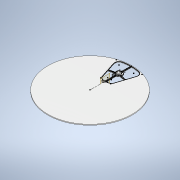
# Autodesk Inventor part: StatorSketches
Saved by Autodesk Inventor 2022.2 (Build 262287000, 287)
## iProperties
Created: 2022-08-10
Part Number: StatorSketches
Material: ABS Plastic
Document SubType Name: Modeling
Designer: ABL
Density: 1.06 g/cm^3
Appearance: Smooth - White
Author: ABL
Autodesk Inventor part; units mm, degrees
ref_plane "YZ Plane" through (0, 0, 0) normal (1, 0, 0) x (0, 1, 0)
ref_plane "XZ Plane" through (0, 0, 0) normal (0, 1, 0) x (-1, 0, 0)
ref_plane "XY Plane" through (0, 0, 0) normal (0, 0, 1) x (1, 0, 0)
sketch "SpoolBorder" plane through (0, 0, 0) normal (0, 0, 1) x (1, 0, 0)
  line L0 (13.9597, -42.9634) -> (26.7564, -82.3478)
  line L1 (0, 0) -> (0, -97.1611) construction
  arc A0 (0, -97.1611) -> (19.2245, -95.2402) centre (0, 0) ccw
  arc A1 (5.3164, -36.0913) -> (0, -35.8603) centre (0, -97.1611) ccw
  arc A2 (19.2245, -95.2402) -> (26.7564, -82.3478) centre (17.2459, -85.4379) ccw
  arc A3 (13.9597, -42.9634) -> (5.3164, -36.0913) centre (4.4491, -46.0536) ccw
  arc A4 (-19.2245, -95.2402) -> (0, -97.1611) centre (0, 0) ccw
  arc A5 (0, -35.8603) -> (-5.3164, -36.0913) centre (0, -97.1611) ccw
  line L2 (-13.9597, -42.9634) -> (-26.7564, -82.3478)
  arc A6 (-26.7564, -82.3478) -> (-19.2245, -95.2402) centre (-17.2459, -85.4379) ccw
  arc A7 (-5.3164, -36.0913) -> (-13.9597, -42.9634) centre (-4.4491, -46.0536) ccw
  point P0 (21.032, -64.73)
  point P1 (30.0244, -92.4057)
  point P2 (12.0397, -37.0542)
  point P3 (-30.0244, -92.4057)
  point P4 (-12.0397, -37.0542)
  dimension "d6" = 97.1611
  dimension "d7" = 10
  dimension "d8" = 10
  dimension "d18" = 61.3008
  dimension "d34" = 10
  measures "d6" distance of L1.start L1.end
  measures "d7" radius of A2
  measures "d8" radius of A3
  measures "d18" distance of L1.end A1.end
  measures "d34" radius of A6
sketch "StatorSpider" plane through (0, 0, 0) normal (0, 0, 1) x (1, 0, 0)
  line L0 (0.0009, -38.9369) -> (0.0009, -97.1369) construction
  line L1 (-3.3991, -69.9999) -> (0.0009, -64.1109) construction
  line L2 (0.0009, -64.1109) -> (3.4009, -69.9999) construction
  line L3 (3.4009, -69.9999) -> (-3.3991, -69.9999) construction
  line L4 (0.0009, -64.1109) -> (3.4997, -62.0909) construction
  arc A0 (3.4997, -62.0909) -> (0.0009, -60.0709) centre (0.0009, -64.1109) ccw
  line L5 (3.4997, -62.0909) -> (6.8997, -67.9799)
  arc A1 (3.4009, -74.0399) -> (6.8997, -67.9799) centre (3.4009, -69.9999) ccw
  line L6 (3.4009, -69.9999) -> (3.4009, -74.0399) construction
  line L7 (3.4009, -69.9999) -> (6.8997, -67.9799) construction
  circle A2 centre (0.0009, -68.0369) radius 4.04
  circle A3 centre (0.0009, -68.0369) radius 1.4 construction
  line L8 (0.0009, -97.1369) -> (0.0009, -35.8361) construction
  line L9 (4.6997, -64.1694) -> (5.6997, -65.9014) construction
  line L10 (3.4009, -74.0399) -> (-3.3991, -74.0399)
  arc A4 (0.0009, -60.0709) -> (-3.4978, -62.0909) centre (0.0009, -64.1109) ccw
  line L11 (0.0009, -64.1109) -> (-3.4978, -62.0909) construction
  line L12 (0.0009, -64.1109) -> (0.0009, -60.0709) construction
  line L13 (-3.4978, -62.0909) -> (-6.8978, -67.9799)
  arc A5 (-6.8978, -67.9799) -> (-3.3991, -74.0399) centre (-3.3991, -69.9999) ccw
  point P0 (1.8944, -62.2189)
  point P1 (0.0009, -69.9999)
  point P2 (5.1997, -65.0354)
  dimension "d11" = 6.8
  dimension "d12" = 4.04
  dimension "d14" = 6.8
  dimension "d15" = 120
  dimension "d16" = 8.08
  dimension "d17" = 2.8
  dimension "d19" = 61.3008
  dimension "d24" = 2
  dimension "d35" = 6.8
  dimension "d36" = 60
  dimension "d37" = 6.8
  measures "d11" distance of L2.end L1.start
  measures "d12" distance of L1.end L4.end
  measures "d14" distance of L4.end L5.end
  measures "d15" angle of L6 L7
  measures "d16" diameter of A2
  measures "d17" diameter of A3
  measures "d19" distance of L0.end L8.end
  measures "d24" distance of L9.start L9.end
  measures "d35" distance of L6.end L10.end
  measures "d36" angle of L12 L11
  measures "d37" distance of L11.end L13.end
sketch "Sketch1" plane through (0, 0, 0) normal (0, 1, 0) x (-1, 0, 0)
  circle A0 centre (0, 0) radius 97.1611
  line L0 (0, 0) -> (0, -99.1611) construction
  circle A1 centre (0, 0) radius 38.9611 construction
  line L1 (0, 0) -> (97.1611, 0) construction
  line L2 (0, 0) -> (33.2311, -91.3016) construction
  line L3 (0, 0) -> (30.0244, -92.4057) construction
  circle A2 centre (0, 0) radius 34.9611 construction
  line L4 (0, -35.8603) -> (11.6517, -35.8603) construction
  line L5 (11.6517, -35.8603) -> (30.0244, -92.4057) construction
  circle A3 centre (0, 0) radius 99.1611
  line L6 (0, 0) -> (-30.0244, -92.4057) construction
  line L7 (0, 0) -> (-33.2311, -91.3016) construction
  line L8 (0, -35.8603) -> (-11.6517, -35.8603) construction
  line L9 (13.9597, -42.9634) -> (26.7564, -82.3478)
  line L10 (0, 0) -> (0, -97.1611) construction
  arc A4 (0, -97.1611) -> (19.2245, -95.2402) centre (0, 0) ccw
  arc A5 (5.3164, -36.0913) -> (0, -35.8603) centre (0, -97.1611) ccw
  arc A6 (19.2245, -95.2402) -> (26.7564, -82.3478) centre (17.2459, -85.4379) ccw
  arc A7 (13.9597, -42.9634) -> (5.3164, -36.0913) centre (4.4491, -46.0536) ccw
  arc A8 (-19.2245, -95.2402) -> (0, -97.1611) centre (0, 0) ccw
  arc A9 (0, -35.8603) -> (-5.3164, -36.0913) centre (0, -97.1611) ccw
  line L11 (-13.9597, -42.9634) -> (-26.7564, -82.3478)
  arc A10 (-26.7564, -82.3478) -> (-19.2245, -95.2402) centre (-17.2459, -85.4379) ccw
  arc A11 (-5.3164, -36.0913) -> (-13.9597, -42.9634) centre (-4.4491, -46.0536) ccw
  line L12 (0, -38.9611) -> (0, -97.1611) construction
  line L13 (-3.4, -70.0241) -> (0, -64.1351) construction
  line L14 (0, -64.1351) -> (3.4, -70.0241) construction
  line L15 (3.4, -70.0241) -> (-3.4, -70.0241) construction
  line L16 (0, -64.1351) -> (3.4987, -62.1151) construction
  arc A12 (3.4987, -62.1151) -> (0, -60.0951) centre (0, -64.1351) ccw
  line L17 (3.4987, -62.1151) -> (6.8987, -68.0041)
  arc A13 (3.4, -74.0641) -> (6.8987, -68.0041) centre (3.4, -70.0241) ccw
  line L18 (3.4, -70.0241) -> (3.4, -74.0641) construction
  line L19 (3.4, -70.0241) -> (6.8987, -68.0041) construction
  circle A14 centre (0, -68.0611) radius 4.04
  circle A15 centre (0, -68.0611) radius 1.4 construction
  line L20 (0, -97.1611) -> (0, -35.8603) construction
  line L21 (4.6987, -64.1936) -> (5.6987, -65.9257) construction
  line L22 (3.4, -74.0641) -> (-3.4, -74.0641)
  arc A16 (0, -60.0951) -> (-3.4987, -62.1151) centre (0, -64.1351) ccw
  line L23 (0, -64.1351) -> (-3.4987, -62.1151) construction
  line L24 (0, -64.1351) -> (0, -60.0951) construction
  line L25 (-3.4987, -62.1151) -> (-6.8987, -68.0041)
  arc A17 (-6.8987, -68.0041) -> (-3.4, -74.0641) centre (-3.4, -70.0241) ccw
  dimension "d0" = 194.3223
  dimension "d1" = 99.1611
  dimension "d2" = 77.9223
  dimension "d3" = 70
  dimension "d4" = 72
  dimension "d5" = 69.9223
  dimension "d29" = 198.3223
  dimension "d32" = 40
  dimension "d33" = 36
  constraints: 18 end point, 5 point on circle, 4 centre point, 4 coincident, 2 horizontal, 2 point on line, 1 perpendicular, 1 vertical, 5 other
  measures "d0" diameter of A0
  measures "d1" distance of L0.start L0.end
  measures "d2" diameter of A1
  measures "d3" angle of L2 L1
  measures "d4" angle of L1 L3
  measures "d5" diameter of A2
  measures "d29" diameter of A3
  measures "d32" angle of L7 L2
  measures "d33" angle of L3 L6
sketch "Sketch2" plane through (0, 0, 0) normal (0, 1, 0) x (-1, 0, 0)
  line L0 (0, 0) -> (0, -97.1611) construction
  line L1 (0, -35.8603) -> (0, -60.0951) construction
  line L2 (0, -97.1611) -> (0, -74.0641) construction
  line L3 (5.1987, -65.0596) -> (6.8987, -68.0041) construction
  line L4 (4.6987, -64.1936) -> (-4.6987, -64.1936) construction
  line L5 (5.6987, -65.9257) -> (-5.6987, -65.9257) construction
  line L6 (0, -35.8603) -> (-1, -35.8603) construction
  line L7 (-1, -35.8603) -> (-1, -35.8685) construction
  line L8 (0, -60.0951) -> (-1, -60.0951) construction
  line L9 (-1, -60.0951) -> (-1, -60.2209) construction
  line L10 (-1, -35.8685) -> (-1, -60.2209)
  line L11 (0, -60.0951) -> (1, -60.0951) construction
  line L12 (1, -60.0951) -> (1, -60.2209) construction
  line L13 (0, -35.8603) -> (1, -35.8603) construction
  line L14 (1, -35.8603) -> (1, -35.8685) construction
  line L15 (1, -35.8685) -> (1, -60.2209)
  line L16 (-1, -74.0641) -> (-1, -97.156)
  line L17 (1, -74.0641) -> (1, -97.156)
  arc A0 (4.6987, -64.1936) -> (19.89, -61.2151) centre (0, 0) ccw
  arc A1 (5.6987, -65.9257) -> (20.4481, -62.9328) centre (0, 0) ccw
  arc A2 (-19.89, -61.2151) -> (-4.6987, -64.1936) centre (0, 0) ccw
  arc A3 (-20.4481, -62.9328) -> (-5.6987, -65.9257) centre (0, 0) ccw
  line L18 (13.9597, -42.9634) -> (26.7564, -82.3478)
  line L19 (0, 0) -> (0, -97.1611) construction
  arc A4 (0, -97.1611) -> (19.2245, -95.2402) centre (0, 0) ccw
  arc A5 (5.3164, -36.0913) -> (0, -35.8603) centre (0, -97.1611) ccw
  arc A6 (19.2245, -95.2402) -> (26.7564, -82.3478) centre (17.2459, -85.4379) ccw
  arc A7 (13.9597, -42.9634) -> (5.3164, -36.0913) centre (4.4491, -46.0536) ccw
  arc A8 (-19.2245, -95.2402) -> (0, -97.1611) centre (0, 0) ccw
  arc A9 (0, -35.8603) -> (-5.3164, -36.0913) centre (0, -97.1611) ccw
  line L20 (-13.9597, -42.9634) -> (-26.7564, -82.3478)
  arc A10 (-26.7564, -82.3478) -> (-19.2245, -95.2402) centre (-17.2459, -85.4379) ccw
  arc A11 (-5.3164, -36.0913) -> (-13.9597, -42.9634) centre (-4.4491, -46.0536) ccw
  line L21 (0, -38.9611) -> (0, -97.1611) construction
  line L22 (-3.4, -70.0241) -> (0, -64.1351) construction
  line L23 (0, -64.1351) -> (3.4, -70.0241) construction
  line L24 (3.4, -70.0241) -> (-3.4, -70.0241) construction
  line L25 (0, -64.1351) -> (3.4987, -62.1151) construction
  arc A12 (3.4987, -62.1151) -> (0, -60.0951) centre (0, -64.1351) ccw
  line L26 (3.4987, -62.1151) -> (6.8987, -68.0041)
  arc A13 (3.4, -74.0641) -> (6.8987, -68.0041) centre (3.4, -70.0241) ccw
  line L27 (3.4, -70.0241) -> (3.4, -74.0641) construction
  line L28 (3.4, -70.0241) -> (6.8987, -68.0041) construction
  circle A14 centre (0, -68.0611) radius 4.04
  circle A15 centre (0, -68.0611) radius 1.4 construction
  line L29 (0, -97.1611) -> (0, -35.8603) construction
  line L30 (4.6987, -64.1936) -> (5.6987, -65.9257) construction
  line L31 (3.4, -74.0641) -> (-3.4, -74.0641)
  arc A16 (0, -60.0951) -> (-3.4987, -62.1151) centre (0, -64.1351) ccw
  line L32 (0, -64.1351) -> (-3.4987, -62.1151) construction
  line L33 (0, -64.1351) -> (0, -60.0951) construction
  line L34 (-3.4987, -62.1151) -> (-6.8987, -68.0041)
  arc A17 (-6.8987, -68.0041) -> (-3.4, -74.0641) centre (-3.4, -70.0241) ccw
  point P0 (-20.4481, -62.9328)
  point P1 (-5.6987, -65.9257)
  point P2 (-4.6987, -64.1936)
  point P3 (5.6987, -65.9257)
  point P4 (20.4481, -62.9328)
  point P5 (19.89, -61.2151)
  point P6 (4.6987, -64.1936)
  dimension "d38" = 1
  dimension "d39" = 1
  dimension "d40" = 1
  dimension "d41" = 1
  dimension "d42" = 2
  constraints: 36 end point, 8 point on circle, 6 point on line, 4 centre point, 4 coincident, 3 horizontal, 3 parallel, 3 vertical, 2 perpendicular, 1 collinear, 24 other
  measures "d38" distance of L1.start L6.end
  measures "d39" distance of L1.end L8.end
  measures "d40" distance of L1.end L11.end
  measures "d41" distance of L1.start L13.end
  measures "d42" distance between parallel lines of L17 L16
extrude "Extrusion1" add sketch "Sketch1" against normal blind 2 contours A0 A6 L9 A7 A5 A9 A11 L11 A10 | A10 L11 A11 A9 A5 A7 L9 A6 A0 | A3 | L17 A13 L22 A17 L25 A16 A12 | A14
ref_plane "Work Plane1" through (0, 0, -35.8603) normal (1, 0, 0) x (0, 1, 0)
sketch "Sketch3" plane through (0, 0, -35.8603) normal (1, 0, 0) x (0, 1, 0)
  circle A0 centre (0, 0) radius 0.005
  point P0 (0, 35.8603)
  dimension "d52" = 0.01
  constraints: 1 centre point
  measures "d52" diameter of A0
sweep "CoilBorder_separation" cut profiles "Sketch3" path "Sketch2" path curves A4 A6 L18 A7 A5 A9 A11 L20 A10 A8
extrude "CoilBorder" cut sketch "Sketch2" against normal up to surface (2 mm away) contours A9 A5 L15 A12 A16 L10 | L10 A16 L34 A2 L20 A11 A9 | A16 A12 L26 A13 L31 A17 L34 | A5 A7 L18 A0 L26 A12 L15 | L34 A3 L20 A2 | L34 A17 L31 L16 A8 A10 L20 A3 | A0 L18 A1 L26 | A1 L18 A6 A4 L17 L31 A13 L26 | L31 L17 A4 A8 L16 | A14
extrude "CoilStatorSpider" add sketch "Sketch2" against normal up to surface (2 mm away) contours A9 A5 L15 A12 A16 L10 | A16 A12 L26 A13 L31 A17 L34 | L34 A3 L20 A2 | A0 L18 A1 L26 | L31 L17 A4 A8 L16 | A14
fillet "StatorSpider_fillet" radius 3 14 edges at (-20.4481, -1.0025, -62.9328) (-19.89, -1.0025, -61.2151) (-4.6987, -1, -64.1936) (-1, -1, -60.2209) (1, -1.0025, -35.8685) (1, -1, -60.2209) (5.6987, -1, -65.9257) (1, -1, -74.0641) (20.4481, -1.0025, -62.9328) (-1, -1, -74.0641) (-5.6987, -1, -65.9257) (19.89, -1.0025, -61.2151) (-1, -1.0025, -35.8685) (4.6987, -1, -64.1936)
fillet "StatorSpider_edgeFillet" radius 1.5 2 edges at (1, -1.0025, -97.156) (-1, -1.0025, -97.156)
extrude "CoilBoltCountersinkOutset" add sketch "Sketch2" along normal blind 2.1 contours A14
fillet "CoilBoltCountersinkOutset_rounding" radius 1 2 edges at (4.04, 0, -68.0611) (4.04, 2.1, -68.0611)
equation "\"d6\" = statorRadius - wallgap"
equation "\"d7\" = coil_cornerRadius"
equation "\"d8\" = d7"
equation "\"d34\" = d7"
equation "\"d11\" = 2 * airgap + statorCoilBolt_diameter + 2 * wallgap"
equation "\"d12\" = 0.5 * d16"
equation "\"d14\" = d11"
equation "\"d16\" = 2 * wallgap + statorCoilBolt_headDiameter + gap"
equation "\"d17\" = statorCoilBolt_diameter + 2 * airgap"
equation "\"d19\" = d18"
equation "\"d24\" = wallgap"
equation "\"d35\" = d11"
equation "\"d37\" = d11"
equation "\"d0\" = -2 * wallgap + 2 * statorRadius"
equation "\"d1\" = statorRadius"
equation "\"d2\" = 2 * driveMagnet_centerSpacingRadius"
equation "\"d4\" = d3 + 0.5 * statorSpokeDegrees"
equation "\"d5\" = -4 * wallgap + 2 * driveMagnet_centerSpacingRadius"
equation "\"d29\" = 2 * statorRadius"
equation "\"d33\" = d32 - statorSpokeDegrees"
equation "\"d30\" = wallgap"
equation "\"d38\" = 0.5 * wallgap"
equation "\"d39\" = 0.5 * wallgap"
equation "\"d40\" = 0.5 * wallgap"
equation "\"d41\" = 0.5 * wallgap"
equation "\"d42\" = wallgap"
equation "\"gap\" = 0.1"
equation "\"airgap\" = 0.4"
equation "\"wallgap\" = 2"
equation "\"driveMagnet_height\" = 5"
equation "\"halbachMagnet_height\" = 3"
equation "\"rotorBandBolt_diameter\" = 2"
equation "\"rotorBandBolt_headDiameter\" = 3.98"
equation "\"rotorBandBolt_headHeight\" = 2"
equation "\"rotorBandHexNut_sideToSide\" = 4"
equation "\"rotorBandHexNut_height\" = 1.2"
equation "\"rotorBandSquareNut_sideLength\" = 4"
equation "\"rotorBandSquareNut_height\" = 1.2"
equation "\"sensorMagnet_diameter\" = 5"
equation "\"sensorMagnet_height\" = 2.66667"
equation "\"sensorMagnet_ringRadius\" = 0.5 * driveMagnet_centerSpacingRadius + 2 * wallgap"
equation "\"rotorRadius\" = 2 * gap + driveMagnet_centerSpacingRadius + driveMagnet_length + wallgap"
equation "\"rotor_mountingLipHeight\" = 0.5 * statorThickness"
equation "\"shaftDiameter\" = 8"
equation "\"flangeBearing_innerDiameter\" = shaftDiameter"
equation "\"flangeBearing_outerDiameter\" = 16"
equation "\"flangeBearing_flangeDiameter\" = 18"
equation "\"flangeBearing_height\" = 5"
equation "\"flangeBearing_flangeHeight\" = 1"
equation "\"coilThickness\" = 12"
equation "\"statorThickness\" = coilThickness + 2 * wallgap"
equation "\"rotorBandThickness\" = wallgap + rotorBandBolt_headHeight + gap"
equation "\"flangeCoupling_innerDiameter\" = shaftDiameter"
equation "\"flangeCoupling_collarOuterDiameter\" = 16"
equation "\"flangeCoupling_flangeDiameter\" = 32"
equation "\"flangeCoupling_flangeHeight\" = 3.1"
equation "\"flangeCoupling_height\" = flangeCoupling_collarHeight + flangeCoupling_flangeHeight"
equation "\"flangeCoupling_mountHoleDiameter\" = 3.9"
equation "\"flangeCoupling_mountHoleEdgeToEdge\" = 2.05"
equation "\"statorRadius\" = driveMagnet_length + driveMagnet_centerSpacingRadius + 2 * gap"
equation "\"statorMountBolt_diameter\" = 4"
equation "\"statorMountBolt_headDiameter\" = 7"
equation "\"statorMountBolt_headHeight\" = 4"
equation "\"statorMountBolt_shaftLength\" = coilThickness + flangeCoupling_flangeHeight + wallgap"
equation "\"statorMountHexNut_sideToSide\" = 8"
equation "\"statorMountHexNut_height\" = 4"
equation "\"coil_percentCoverage\" = 0.6"
equation "\"statorSpokeDegrees\" = 4deg"
equation "\"coil_cornerRadius\" = 10"
equation "\"statorCoilBolt_diameter\" = 2"
equation "\"statorCoilBolt_headDiameter\" = 3.98"
equation "\"statorCoilBolt_headHeight\" = 2"
equation "\"statorCoilBolt_shaftLength\" = coilThickness"
equation "\"statorCoilHexNut_sideToSide\" = 4"
equation "\"statorCoilHexNut_height\" = 1.2"
equation "\"driveMagnet_centerSpacingRadius\" = 38.96113"
equation "\"driveMagnet_length\" = 60"
equation "\"flangeCoupling_collarHeight\" = 10"
body "Solid1"
